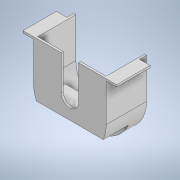
# Autodesk Inventor part: TapaEje
Saved by Autodesk Inventor 2020 (Build 240168000, 168)
## iProperties
Created: 2019-11-12
Part Number: TapaEje
Material: Genérico
Document SubType Name: Modeling
Designer: Usuario
Density: 1 g/cm^3
Appearance: Valor por defecto
Author: Usuario
## iProperties of the stored document _3DPrint.ipt
Created: 2019-11-12
Part Number: _3DPrint
Material: Genérico
Document SubType Name: Modeling
Designer: Usuario
Density: 1 g/cm^3
Appearance: Valor por defecto
Author: Usuario
Autodesk Inventor part; units mm, degrees
ref_plane "YZ Plane" through (0, 0, 0) normal (1, 0, 0) x (0, 1, 0)
ref_plane "XZ Plane" through (0, 0, 0) normal (0, 1, 0) x (-1, 0, 0)
ref_plane "XY Plane" through (0, 0, 0) normal (0, 0, 1) x (1, 0, 0)
sketch "Boceto1" plane through (0, 0, 0) normal (0, 0, 1) x (1, 0, 0)
  arc A0 (-52.25, 0) -> (52.25, 0) centre (0, 0) ccw
  line L0 (-52.25, 0) -> (-52.25, 57.25)
  line L1 (-52.25, 57.25) -> (-49.25, 57.25)
  line L2 (52.25, 57.25) -> (52.25, 0)
  arc A1 (52.25, 0) -> (-52.25, 0) centre (0, 0) ccw construction
  line L3 (0, -52.25) -> (0, 57.25) construction
  line L4 (-49.25, 57.25) -> (-49.25, 0)
  arc A2 (-49.25, 0) -> (49.25, 0) centre (0, 0) ccw
  line L5 (49.25, 0) -> (49.25, 57.25)
  line L6 (49.25, 57.25) -> (-49.25, 57.25) construction
  line L7 (49.25, 57.25) -> (49.25, 57.25)
  line L8 (-49.25, 57.25) -> (-49.25, 57.25)
  line L9 (-49.25, 57.25) -> (0, 57.25) construction
  line L10 (0, 57.25) -> (49.25, 57.25) construction
  line L11 (49.25, 57.25) -> (52.25, 57.25)
  dimension "d0" = 104.5
  dimension "d2" = 109.5
  dimension "d3" = 3
  constraints: 24 end point, 9 perpendicular, 7 point on circle, 3 centre point, 2 point on line, 2 tangent, 2 vertical, 1 coincident, 1 collinear, 1 parallel, 2 other
  measures "d0" diameter of A0
  measures "d2" distance of L3.start L3.end
  measures "d3" distance between parallel lines of L0 L4
extrude "Extrusión1" add sketch "Boceto1" along normal blind 10
sketch "Boceto2" plane through (0, 0, 10) normal (0, 0, 1) x (1, 0, 0)
  line L0 (49.25, 57.25) -> (49.25, 0) projected
  arc A0 (-49.25, 0) -> (49.25, 0) centre (0, 0) ccw projected
  line L1 (-49.25, 0) -> (-49.25, 57.25) projected
  line L2 (-49.25, 57.25) -> (-52.25, 57.25) projected
  line L3 (-52.25, 57.25) -> (-52.25, 0) projected
  arc A1 (-52.25, 0) -> (52.25, 0) centre (0, 0) ccw projected
  line L4 (52.25, 0) -> (52.25, 57.25) projected
  line L5 (52.25, 57.25) -> (49.25, 57.25) projected
  line L6 (-49.25, 57.25) -> (-52.25, 57.25) projected
  line L7 (-52.25, 57.25) -> (-67.25, 57.25)
  line L8 (-67.25, 57.25) -> (-67.25, 54.25)
  line L9 (-67.25, 54.25) -> (-52.25, 54.25)
  line L10 (-52.25, 54.25) -> (-52.25, 57.25)
  line L11 (52.25, 57.25) -> (49.25, 57.25) projected
  line L12 (52.25, 57.25) -> (67.25, 57.25)
  line L13 (67.25, 57.25) -> (67.25, 54.25)
  line L14 (67.25, 54.25) -> (52.25, 54.25)
  line L15 (52.25, 54.25) -> (52.25, 57.25)
  point P0 (49.5, 57.5)
  dimension "d6" = 15
  dimension "d7" = 3
  dimension "d8" = 15
  dimension "d9" = 3
  constraints: 16 end point, 4 parallel, 2 horizontal, 2 perpendicular, 1 other
  measures "d6" distance of L2.end L7.end
  measures "d7" distance of L7.end L8.end
  measures "d8" distance of L4.end L12.end
  measures "d9" distance of L12.end L13.end
extrude "Extrusión3" add sketch "Boceto2" along normal blind 9
sketch "Boceto3" plane through (0, 0, 19) normal (0, 0, 1) x (1, 0, 0)
  line L0 (-52.25, 54.25) -> (-52.25, 0) projected
  line L1 (-49.25, 0) -> (-49.25, 57.25) projected
  line L2 (-49.25, 57.25) -> (-67.25, 57.25) projected
  line L3 (-67.25, 54.25) -> (-52.25, 54.25) projected
  line L4 (-67.25, 57.25) -> (-67.25, 54.25) projected
  line L5 (49.25, 57.25) -> (49.25, 0) projected
  line L6 (52.25, 0) -> (52.25, 54.25) projected
  line L7 (52.25, 54.25) -> (67.25, 54.25) projected
  line L8 (67.25, 54.25) -> (67.25, 57.25) projected
  line L9 (67.25, 57.25) -> (49.25, 57.25) projected
  arc A0 (-52.25, 0) -> (52.25, 0) centre (0, 0) ccw construction
  line L10 (-47.9531, -20.75) -> (47.9531, -20.75)
  arc A1 (-52.25, 0) -> (-47.9531, -20.75) centre (0, 0) ccw
  arc A2 (47.9531, -20.75) -> (52.25, 0) centre (0, 0) ccw
  arc A3 (-49.25, 0) -> (-45.9402, -17.75) centre (0, 0) ccw
  arc A4 (44.6654, -20.75) -> (45.9402, -17.75) centre (0, 0) ccw construction
  line L11 (-49.1426, -17.75) -> (-45.9402, -17.75) construction
  arc A5 (-45.9402, -17.75) -> (-44.6654, -20.75) centre (0, 0) ccw construction
  line L12 (-45.9402, -17.75) -> (45.9402, -17.75)
  arc A6 (45.9402, -17.75) -> (49.25, 0) centre (0, 0) ccw
  line L13 (45.9402, -17.75) -> (49.1426, -17.75) construction
  dimension "d14" = 78
  dimension "d15" = 3
  constraints: 17 point on circle, 10 end point, 6 centre point, 4 point on line, 2 coincident, 1 horizontal, 1 parallel
  measures "d14" distance between parallel lines of L9 L10
  measures "d15" distance between parallel lines of L10 L11
extrude "Extrusión4" add sketch "Boceto3" along normal blind 39
sketch "Boceto4" plane through (0, 0, 19) normal (0, 0, 1) x (1, 0, 0)
  arc A0 (-47.9531, -20.75) -> (47.9531, -20.75) centre (0, 0) ccw projected
  line L0 (-47.9531, -20.75) -> (47.9531, -20.75) projected
extrude "Extrusión5" add sketch "Boceto4" along normal blind 3
sketch "Boceto5" plane through (0, 0, 58) normal (0, 0, 1) x (1, 0, 0)
  line L0 (-52.25, 54.25) -> (-52.25, 0) projected
  arc A0 (-52.25, 0) -> (-47.9531, -20.75) centre (0, 0) ccw projected
  line L1 (-47.9531, -20.75) -> (47.9531, -20.75) projected
  arc A1 (47.9531, -20.75) -> (52.25, 0) centre (0, 0) ccw projected
  line L2 (52.25, 0) -> (52.25, 54.25) projected
  line L3 (-52.25, 57.25) -> (-52.25, 0) projected
  line L4 (-52.25, 54.25) -> (-52.25, 57.25)
  line L5 (-52.25, 57.25) -> (-12.5, 57.25)
  line L6 (-12.5, 57.25) -> (-12.5, 7.25)
  line L7 (0, -5.25) -> (0, -5.25)
  line L8 (12.5, 7.25) -> (12.5, 57.25)
  line L9 (12.5, 57.25) -> (52.25, 57.25)
  line L10 (52.25, 57.25) -> (52.25, 54.25)
  arc A2 (-12.5, 7.25) -> (0, -5.25) centre (0, 7.25) ccw
  arc A3 (0, -5.25) -> (12.5, 7.25) centre (0, 7.25) ccw
  point P0 (-12.5, -5.25)
  point P1 (12.5, -5.25)
  point P2 (0, -5.25)
  dimension "d20" = 25
  dimension "d22" = 12.5
  dimension "d23" = 12.5
  dimension "d24" = 50
  constraints: 14 end point, 6 point on line, 5 perpendicular, 4 point on circle, 4 tangent, 2 centre point, 1 concentric, 1 vertical
  measures "d20" distance of point (-12.5, -5.25) point (12.5, -5.25)
  measures "d22" distance from line of L6 point (0, 0)
  measures "d23" radius of A2
  measures "d24" distance from line of L9 A2.centre
extrude "Extrusión6" add sketch "Boceto5" against normal blind 3
